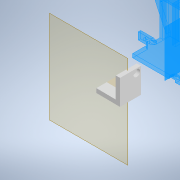
# Autodesk Inventor part: gira  down
Saved by Autodesk Inventor 2020 (Build 240168000, 168)
## iProperties
Created: 2023-03-26
Part Number: gira  down
Material: Generic
Document SubType Name: Modeling
Designer: super
Density: 1 g/cm^3
Appearance: Default
Author: super
Autodesk Inventor part; units mm, degrees
ref_plane "YZ Plane" through (0, 0, 0) normal (1, 0, 0) x (0, 1, 0)
ref_plane "XZ Plane" through (0, 0, 0) normal (0, 1, 0) x (-1, 0, 0)
ref_plane "XY Plane" through (0, 0, 0) normal (0, 0, 1) x (1, 0, 0)
ref_plane "Work Plane1" through (45.1487, 198.4118, 0) normal (0, 0, 1) x (-1, 0, 0)
sketch "Sketch1" plane through (45.1487, 198.4118, 0) normal (0, 0, 1) x (-1, 0, 0)
  line L0 (-15.0122, 14.6271) -> (-15.0122, 74.6271)
  line L1 (-15.0122, 74.6271) -> (41.5559, 74.0451)
  line L2 (41.5559, 64.0446) -> (-5.0122, 64.5237)
  line L3 (-5.0122, 64.5237) -> (-5.0122, 14.6271)
  line L4 (-15.0122, 14.6271) -> (-5.0122, 14.6271)
  line L5 (41.5559, 64.0446) -> (41.5559, 74.0451)
  point P0 (45.1487, 198.4118)
  dimension "d1" = 10
  dimension "d13" = 60
  constraints: 12 end point, 1 horizontal, 1 perpendicular, 1 vertical, 1 other
  measures "d1" distance between parallel lines of L1 L2
  measures "d13" distance of L0.start L0.end
extrude "Extrusion1" add sketch "Sketch1" along normal mid plane 50
sketch "Sketch2" plane through (60.1609, 123.7848, 25) normal (1, 0, 0) x (0, 0, -1)
  line L0 (50, 60) -> (50, 0) projected
  line L1 (0, 60) -> (50, 60) projected
  point P0 (40, 50)
  dimension "d11" = 10
  dimension "d12" = 10
  measures "d11" distance from line of L0 point (40, 50)
  measures "d12" distance from line of L1 point (40, 50)
hole "Hole1" at (60.1609, 173.7848, -15) direction (-1, 0, 0) diameter 6.6 depth 10 counterbore diameter 16 counterbore depth 8
body "Solid1"
